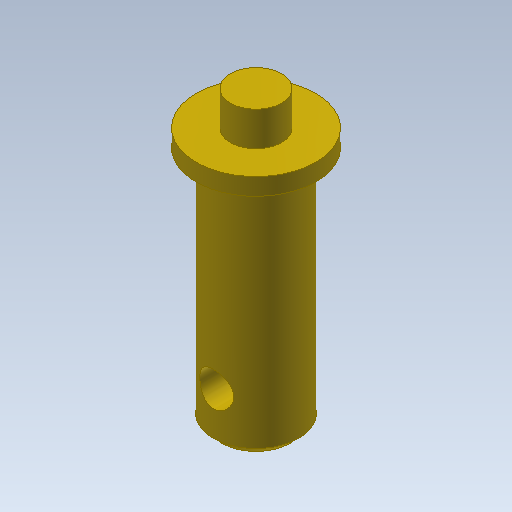
# Autodesk Inventor part: Locking Pin
Saved by Autodesk Inventor 2020 (Build 240168000, 168)
## iProperties
Created: 2012-11-06
Part Number: Locking Pin
Document SubType Name: Modeling
Designer: Lance
Density: 1 g/cm^3
Material: Generic
Appearance: Glossy - Gold
Author: Lance
Autodesk Inventor part; units mm, degrees
ref_plane "YZ Plane" through (0, 0, 0) normal (1, 0, 0) x (0, 1, 0)
ref_plane "XZ Plane" through (0, 0, 0) normal (0, 1, 0) x (-1, 0, 0)
ref_plane "XY Plane" through (0, 0, 0) normal (0, 0, 1) x (1, 0, 0)
sketch "Sketch1" plane through (0, 0, 0) normal (0, 0, 1) x (1, 0, 0)
  line L0 (0, 8.5) -> (0, -8.5)
  line L1 (0, -8.5) -> (2.5, -8.5)
  line L2 (2.5, -8.5) -> (2.5, 5.5)
  line L3 (2.5, 5.5) -> (3.5, 5.5)
  line L4 (3.5, 5.5) -> (3.5, 6.5)
  line L5 (3.5, 6.5) -> (1.5, 6.5)
  line L6 (1.5, 6.5) -> (1.5, 8.5)
  line L7 (1.5, 8.5) -> (0, 8.5)
  point P0 (0, 0)
  point P1 (0, 0)
  dimension "d0" = 3
  dimension "d1" = 5
  dimension "d2" = 7
  dimension "d3" = 2
  dimension "d4" = 1
  dimension "d5" = 17
  constraints: 16 end point, 5 parallel, 2 perpendicular, 1 coincident, 1 midpoint, 1 vertical
  measures "d0" diameter of L6 L0
  measures "d1" diameter of L2 L0
  measures "d2" diameter of L4 L0
  measures "d3" distance between parallel lines of L5 L7
  measures "d4" distance between parallel lines of L3 L5
  measures "d5" distance between parallel lines of L1 L7
revolve "Revolution1" add sketch "Sketch1" angle 360 about axis through (0, 8.5, 0) along (0, -1, 0)
sketch "Sketch2" plane through (0, 0, 0) normal (0, 0, 1) x (1, 0, 0)
  circle A0 centre (0, -5.5) radius 1
  line L0 (-2.5, -8.5) -> (2.5, -8.5) projected
  point P0 (0, 0)
  point P1 (0, -8.5)
  dimension "d7" = 2
  dimension "d8" = 4
  constraints: 1 centre point, 1 midpoint, 1 vertical alignment
  measures "d7" diameter of A0
extrude "Extrusion1" cut sketch "Sketch2" along normal through all both and the other way through all
chamfer "Chamfer1" distance 0.5 angle 45 1 edges at (-2.5, -8.5, 0)
body "Solid1"
